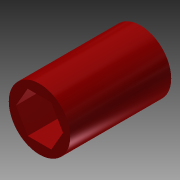
# Autodesk Inventor part: Carriage Spacer - Upper
Saved by Autodesk Inventor 2013 (Build 170138000, 138)
## iProperties
Created: 2013-04-02
Part Number: Carriage Spacer - Upper
Material: Generic
Document SubType Name: Modeling
Designer: mvarma
Density: 1 g/cm^3
Author: mvarma
Autodesk Inventor part; units mm, degrees
ref_plane "YZ Plane" through (0, 0, 0) normal (1, 0, 0) x (0, 1, 0)
ref_plane "XZ Plane" through (0, 0, 0) normal (0, 1, 0) x (-1, 0, 0)
ref_plane "XY Plane" through (0, 0, 0) normal (0, 0, 1) x (1, 0, 0)
sketch "Sketch1" plane through (0, 0, 0) normal (0, 0, 1) x (1, 0, 0)
  circle A0 centre (0, 0) radius 7.1437
  line L0 (-5.4993, 0) -> (-2.7496, 4.7625)
  line L1 (-2.7496, 4.7625) -> (2.7496, 4.7625)
  line L2 (2.7496, 4.7625) -> (5.4993, 0)
  line L3 (5.4993, 0) -> (2.7496, -4.7625)
  line L4 (2.7496, -4.7625) -> (-2.7496, -4.7625)
  line L5 (-2.7496, -4.7625) -> (-5.4993, 0)
  dimension "d0" = 9.525
  dimension "d1" = 14.2875
  constraints: 12 end point, 2 coincident, 1 centre point, 1 horizontal, 13 other
  measures "d0" distance between parallel lines of L4 L1
  measures "d1" diameter of A0
extrude "Extrusion1" add sketch "Sketch1" along normal blind 23.5204
body "Solid1"
